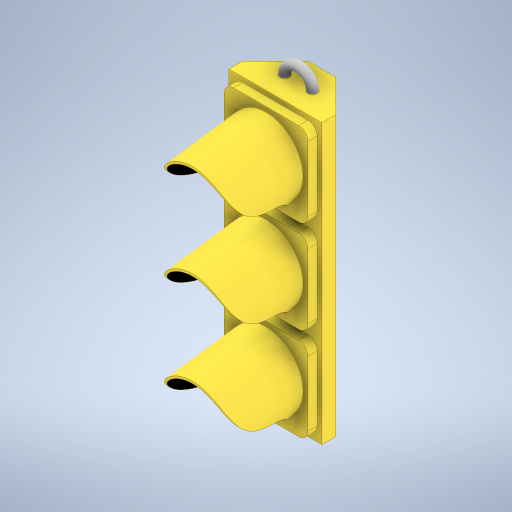
# Autodesk Inventor part: light
Saved by Autodesk Inventor 2024 (Build 280153000, 153)
## iProperties
Created: 2023-10-09
Part Number: light
Material: Generic
Document SubType Name: Modeling
Designer: Raina
Density: 1 g/cm^3
Appearance: Default
Author: Raina
Autodesk Inventor part; units mm, degrees
ref_plane "YZ Plane" through (0, 0, 0) normal (1, 0, 0) x (0, 1, 0)
ref_plane "XZ Plane" through (0, 0, 0) normal (0, 1, 0) x (-1, 0, 0)
ref_plane "XY Plane" through (0, 0, 0) normal (0, 0, 1) x (1, 0, 0)
sketch "Sketch1" plane through (0, 0, 0) normal (0, 0, 1) x (1, 0, 0)
  line L0 (0, 0) -> (292.1, 0) construction
  line L1 (292.1, 0) -> (292.1, 762) construction
  line L2 (292.1, 762) -> (0, 762) construction
  line L3 (0, 762) -> (0, 0) construction
  line L4 (0, 762) -> (254, 762)
  line L5 (254, 762) -> (254, 0)
  line L6 (254, 0) -> (0, 0)
  line L7 (0, 0) -> (0, 762)
  dimension "d0" = 292.1
  dimension "d1" = 762
  dimension "d2" = 254
  constraints: 16 end point, 4 parallel, 2 horizontal, 2 perpendicular, 1 point on line
  measures "d0" distance of L2.end L1.end
  measures "d1" distance of L1.end L0.end
  measures "d2" distance of L5.end L6.end
extrude "Extrusion1" add sketch "Sketch1" along normal blind 152.4
sketch "Sketch2" plane through (0, 0, 152.4) normal (0, 0, 1) x (1, 0, 0)
  line L0 (0, 508) -> (254, 508)
  line L1 (0, 762) -> (0, 0) projected
  line L2 (0, 254) -> (254, 254)
  line L3 (254, 0) -> (254, 762) projected
  constraints: 4 end point, 3 point on line, 2 horizontal
sketch "Sketch3" plane through (0, 0, 152.4) normal (0, 0, 1) x (1, 0, 0)
  line L0 (254, 762) -> (0, 762) projected
  line L1 (127, 762) -> (127, 736.5989) construction
  line L2 (127, 736.5989) -> (0, 736.5989) construction
  line L3 (0, 762) -> (0, 0) projected
  line L4 (127, 508) -> (127, 482.6) construction
  line L5 (127, 482.6) -> (0, 482.6) construction
  line L6 (127, 254) -> (127, 228.6) construction
  line L7 (127, 228.6) -> (0, 228.6) construction
  dimension "d11" = 25.4
  dimension "d12" = 25.4
  constraints: 12 end point, 4 perpendicular, 3 point on line, 2 vertical, 1 midpoint
  measures "d11" distance of L4.start L4.end
  measures "d12" distance of L6.start L6.end
sketch "Sketch5" plane through (0, 0, 152.4) normal (0, 0, 1) x (1, 0, 0)
  circle A0 centre (127, 127) radius 101.6
  circle A1 centre (127, 127) radius 95.25
  circle A2 centre (127, 381) radius 101.6
  circle A3 centre (127, 381) radius 95.25
  circle A4 centre (127, 635) radius 101.6
  circle A5 centre (127, 635) radius 95.25
  point P0 (0, 0)
  dimension "d17" = 203.2
  dimension "d18" = 190.5
  dimension "d19" = 203.2
  dimension "d20" = 190.5
  dimension "d21" = 203.2
  dimension "d22" = 190.5
  constraints: 6 centre point, 3 coincident
  measures "d17" diameter of A0
  measures "d18" diameter of A1
  measures "d19" diameter of A2
  measures "d20" diameter of A3
  measures "d21" diameter of A4
  measures "d22" diameter of A5
sketch "Sketch4" plane through (0, 0, 0) normal (-1, 0, 0) x (0, 0, 1)
  line L0 (152.4, 0) -> (152.4, 762) projected
  line L1 (152.4, 482.6) -> (0, 482.6) construction
  line L2 (0, 762) -> (0, 0) projected
  line L3 (152.4, 228.6) -> (0, 228.6) construction
  line L4 (152.4, 762) -> (152.4, 0) projected
  line L5 (152.4, 635) -> (353.6225, 606.72)
  line L6 (152.4, 635) -> (355.6, 635) construction
  line L7 (152.4, 381) -> (353.6225, 352.72)
  line L8 (152.4, 381) -> (355.6, 381) construction
  line L9 (152.4, 127) -> (353.6225, 98.72)
  line L10 (152.4, 127) -> (355.6, 127) construction
  dimension "d23" = 203.2
  dimension "d24" = 8
  dimension "d25" = 203.2
  dimension "d26" = 8
  dimension "d27" = 203.2
  dimension "d28" = 8
  constraints: 16 end point, 6 point on line, 4 horizontal, 3 equal length, 1 midpoint, 1 perpendicular
  measures "d23" distance of L5.start L5.end
  measures "d24" angle of L5 L6
  measures "d25" distance of L7.start L7.end
  measures "d26" angle of L7 L8
  measures "d27" distance of L9.start L9.end
  measures "d28" angle of L9 L10
sweep "Sweep1" add profiles "Sketch5" path "Sketch4" path curves L5 contours A4
sweep "Sweep2" add profiles "Sketch5" path "Sketch4" path curves L7 contours A2
sweep "Sweep3" add profiles "Sketch5" path "Sketch4" path curves L9 contours A0
sketch "Sketch6" plane through (254, 0, 0) normal (1, 0, 0) x (0, 0, -1)
  line L0 (0, 0) -> (-152.4, 0) projected
  line L1 (-152.4, 0) -> (-152.4, 762) projected
  line L2 (0, 0) -> (-152.4, 0)
  line L3 (-152.4, 0) -> (-152.4, 254)
  line L4 (-152.4, 254) -> (0, 254)
  line L5 (0, 254) -> (0, 0)
  line L6 (0, 254) -> (-152.4, 254)
  line L7 (-152.4, 254) -> (-152.4, 508)
  line L8 (-152.4, 508) -> (0, 508)
  line L9 (0, 508) -> (0, 254)
  line L10 (0, 508) -> (-152.4, 508)
  line L11 (-152.4, 508) -> (-152.4, 762)
  line L12 (-152.4, 762) -> (0, 762)
  line L13 (0, 762) -> (0, 508)
  line L14 (-353.6225, 200.32) -> (-353.6225, -2.88) projected
  line L15 (-353.6225, 200.32) -> (-353.6225, 98.72)
  arc A0 (-353.6225, 200.32) -> (-286.3782, 98.7561) centre (-243.3006, 200.32) ccw
  line L16 (-152.4, 98.72) -> (-152.4, 0)
  arc A1 (-152.4, 0) -> (-217.0291, 84.3999) centre (-239.824, 0) ccw
  arc A2 (-286.3782, 98.7561) -> (-217.0291, 84.3999) centre (-215.7421, 265.2946) ccw
  line L17 (-152.4, 0) -> (-353.6225, -2.88)
  line L18 (-353.6225, -2.88) -> (-353.6225, 200.32)
  arc A3 (-353.6225, 454.32) -> (-286.3782, 352.7561) centre (-243.3006, 454.32) ccw
  arc A4 (-152.4, 254) -> (-217.0291, 338.3999) centre (-239.824, 254) ccw
  arc A5 (-286.3782, 352.7561) -> (-217.0291, 338.3999) centre (-215.7421, 519.2946) ccw
  line L19 (-152.4, 254) -> (-353.6225, 251.12)
  line L20 (-353.6225, 251.12) -> (-353.6225, 454.32)
  arc A6 (-353.6225, 708.32) -> (-286.3782, 606.7561) centre (-243.3006, 708.32) ccw
  arc A7 (-152.4, 508) -> (-217.0291, 592.3999) centre (-239.824, 508) ccw
  arc A8 (-286.3782, 606.7561) -> (-217.0291, 592.3999) centre (-215.7421, 773.2946) ccw
  line L21 (-152.4, 508) -> (-353.6225, 505.12)
  line L22 (-353.6225, 505.12) -> (-353.6225, 708.32)
  arc A9 (-353.6225, 200.32) -> (-286.3782, 98.7561) centre (-243.3006, 200.32) ccw
  arc A10 (-152.4, 0) -> (-217.0291, 84.3999) centre (-239.824, 0) ccw
  arc A11 (-286.3782, 98.7561) -> (-217.0291, 84.3999) centre (-215.7421, 265.2946) ccw
  line L23 (-152.4, 0) -> (-353.6225, -2.88)
  line L24 (-353.6225, -2.88) -> (-353.6225, 200.32)
  dimension "d38" = 101.6
  constraints: 44 end point, 24 point on circle, 12 centre point, 10 tangent, 6 parallel, 3 horizontal, 3 perpendicular, 3 point on line, 2 collinear, 1 midpoint
  measures "d38" distance of L14.start L15.end
extrude "Extrusion2" cut sketch "Sketch6" against normal blind 776.2875 contours L17 L14 A0 A2 A1 | L19 L20 A3 A5 A4 | L21 L22 A6 A8 A7
sketch "Sketch7" plane through (0, 0, 152.4) normal (0, 0, 1) x (1, 0, 0)
  circle A0 centre (127, 127) radius 95.25 projected
  circle A1 centre (127, 127) radius 101.6 projected
  circle A2 centre (127, 381) radius 101.6 projected
  circle A3 centre (127, 635) radius 101.6 projected
  line L0 (0, 0) -> (0, 762) projected
  line L1 (0, 762) -> (254, 762) projected
  line L2 (254, 762) -> (254, 0) projected
  line L3 (254, 0) -> (0, 0) projected
  circle A4 centre (127, 381) radius 95.25 projected
  circle A5 centre (127, 635) radius 95.25 projected
  line L4 (38.1, 520.7) -> (215.9, 520.7)
  line L5 (241.3, 546.1) -> (241.3, 723.9)
  line L6 (215.9, 749.3) -> (38.1, 749.3)
  line L7 (12.7, 723.9) -> (12.7, 546.1)
  line L8 (38.1, 12.7) -> (215.9, 12.7)
  line L9 (241.3, 38.1) -> (241.3, 215.9)
  line L10 (215.9, 241.3) -> (38.1, 241.3)
  line L11 (12.7, 215.9) -> (12.7, 38.1)
  line L12 (38.1, 266.7) -> (215.9, 266.7)
  line L13 (241.3, 292.1) -> (241.3, 469.9)
  line L14 (215.9, 495.3) -> (38.1, 495.3)
  line L15 (12.7, 469.9) -> (12.7, 292.1)
  arc A6 (38.1, 495.3) -> (12.7, 469.9) centre (38.1, 469.9) ccw
  arc A7 (241.3, 469.9) -> (215.9, 495.3) centre (215.9, 469.9) ccw
  arc A8 (215.9, 266.7) -> (241.3, 292.1) centre (215.9, 292.1) ccw
  arc A9 (12.7, 292.1) -> (38.1, 266.7) centre (38.1, 292.1) ccw
  arc A10 (38.1, 241.3) -> (12.7, 215.9) centre (38.1, 215.9) ccw
  arc A11 (215.9, 12.7) -> (241.3, 38.1) centre (215.9, 38.1) ccw
  arc A12 (241.3, 215.9) -> (215.9, 241.3) centre (215.9, 215.9) ccw
  arc A13 (12.7, 38.1) -> (38.1, 12.7) centre (38.1, 38.1) ccw
  arc A14 (12.7, 546.1) -> (38.1, 520.7) centre (38.1, 546.1) ccw
  arc A15 (215.9, 520.7) -> (241.3, 546.1) centre (215.9, 546.1) ccw
  arc A16 (38.1, 749.3) -> (12.7, 723.9) centre (38.1, 723.9) ccw
  arc A17 (241.3, 723.9) -> (215.9, 749.3) centre (215.9, 723.9) ccw
  point P0 (241.3, 749.3)
  point P1 (241.3, 520.7)
  point P2 (12.7, 749.3)
  point P3 (241.3, 241.3)
  point P4 (241.3, 12.7)
  point P5 (241.3, 495.3)
  point P6 (241.3, 266.7)
  dimension "d41" = 228.6
  dimension "d42" = 228.6
  dimension "d43" = 228.6
  dimension "d44" = 228.6
  dimension "d45" = 25.4
  constraints: 24 end point, 24 point on circle, 24 tangent, 14 point on line, 12 centre point, 11 equal radius, 6 parallel, 3 horizontal, 3 perpendicular
  measures "d41" distance of point (12.7, 749.3) point (241.3, 749.3)
  measures "d42" distance of point (241.3, 749.3) point (241.3, 520.7)
  measures "d43" distance of point (241.3, 241.3) point (241.3, 12.7)
  measures "d44" distance of point (241.3, 495.3) point (241.3, 266.7)
  measures "d45" radius of A6
extrude "Extrusion3" cut sketch "Sketch7" against normal blind 25.4 contours L0 L1 L2 L3
sketch "Sketch8" plane through (0, 762, 0) normal (0, 1, 0) x (1, 0, 0)
  line L0 (0, 0) -> (0, -127) projected
  line L1 (0, -88.9) -> (88.9, 0)
  line L2 (0, -88.9) -> (203.2, -88.9) construction
  line L3 (254, -127) -> (0, -127) projected
  line L4 (0, -127) -> (0, 0) projected
  line L5 (0, 0) -> (254, 0) projected
  line L6 (254, 0) -> (254, -127) projected
  line L7 (254, -127) -> (0, -127) projected
  line L8 (0, -127) -> (0, 0) projected
  line L9 (0, 0) -> (254, 0) projected
  line L10 (254, 0) -> (254, -127) projected
  line L11 (254, -88.9) -> (165.1, 0)
  line L12 (254, -88.9) -> (410.0102, -88.9) construction
  line L13 (254, 0) -> (0, 0) projected
  line L14 (88.9, 0) -> (165.1, 0)
  dimension "d49" = 45
  dimension "d50" = 135
  constraints: 10 end point, 5 point on line, 2 horizontal
  measures "d49" angle of L2 L1
  measures "d50" angle of L12 L11
extrude "Extrusion4" cut sketch "Sketch8" against normal through all contours L5 L1 L0 | L5 L6 L11
sketch "Sketch9" plane through (0, 762, 127) normal (0, 1, 0) x (1, 0, 0)
  line L0 (215.9, 0) -> (38.1, 0) projected
  line L1 (127, 0) -> (127, 127) construction
  line L2 (88.9, 127) -> (165.1, 127) projected
  line L3 (165.1, 63.5) -> (88.9, 63.5) construction
  circle A0 centre (88.9, 63.5) radius 12.7
  circle A1 centre (165.1, 63.5) radius 12.7
  point P0 (0, 127)
  dimension "d53" = 25.4
  dimension "d54" = 25.4
  constraints: 4 end point, 2 centre point, 2 coincident, 2 midpoint
  measures "d53" diameter of A0
  measures "d54" diameter of A1
revolve "Revolution1" add sketch "Sketch9" angle 180 about axis through (127, 762, 127) along (0, 0, -1) contours A0
sketch "Sketch11" plane through (12.7, 546.1, 152.4) normal (-1, 0, 0) x (0, 0, 1)
  line L0 (-25.4, -508) -> (-25.4, -330.2) projected
  line L1 (-25.4, -419.1) -> (0, -419.1) construction
  line L2 (0, -514.35) -> (0, -323.85) projected
  line L3 (-12.7, -419.1) -> (-12.7, -508) construction
  line L4 (0, -508) -> (-25.4, -508) projected
  line L5 (-12.7, -330.2) -> (-12.7, -419.1) construction
  circle A0 centre (-12.7, -374.65) radius 6.35
  circle A1 centre (-12.7, -463.55) radius 6.35
  circle A2 centre (-12.7, -120.65) radius 6.35
  circle A3 centre (-12.7, -209.55) radius 6.35
  circle A4 centre (-12.7, 133.35) radius 6.35
  circle A5 centre (-12.7, 44.45) radius 6.35
  point P0 (-152.4, -546.1)
  dimension "d58" = 12.7
  dimension "d59" = 12.7
  dimension "d60" = 12.7
  dimension "d61" = 12.7
  dimension "d62" = 12.7
  dimension "d63" = 12.7
  constraints: 6 centre point, 6 end point, 6 midpoint, 1 perpendicular, 1 point on line
  measures "d58" diameter of A0
  measures "d59" diameter of A1
  measures "d60" diameter of A2
  measures "d61" diameter of A3
  measures "d62" diameter of A4
  measures "d63" diameter of A5
sketch "Sketch12" plane through (12.7, 546.1, 152.4) normal (-1, 0, 0) x (0, 0, 1)
  line L0 (0, 177.8) -> (-25.4, 177.8) projected
  line L1 (-25.4, 0) -> (-25.4, 177.8) projected
  line L2 (-25.4, 177.8) -> (-25.4, 0)
  point P0 (-152.4, -546.1)
  constraints: 2 end point, 1 vertical
revolve "Revolution2" add sketch "Sketch11" angle 180 about axis through (12.7, 723.9, 127) along (0, -1, 0)
body "Solid1"
